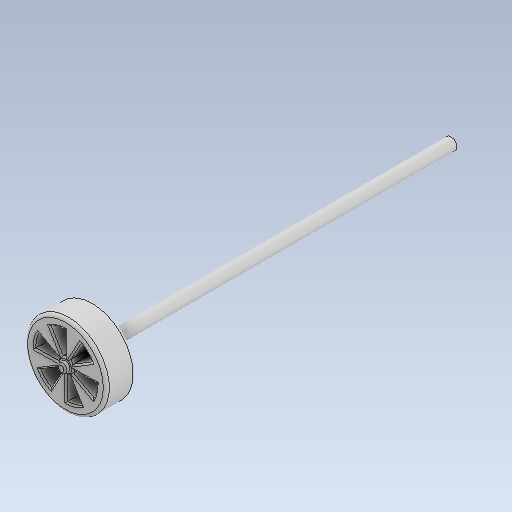
# Autodesk Inventor part: WHEEL 2_CPY1
Saved by Autodesk Inventor 2021 (Build 250183000, 183)
## iProperties
Created: 2021-07-08
Part Number: WHEEL 2_CPY1
Material: Generic
Document SubType Name: Modeling
Designer: HP
Density: 1 g/cm^3
Appearance: Default
Author: AKSHATA
Autodesk Inventor part; units mm, degrees
ref_plane "YZ Plane" through (0, 0, 0) normal (1, 0, 0) x (0, 1, 0)
ref_plane "XZ Plane" through (0, 0, 0) normal (0, 1, 0) x (-1, 0, 0)
ref_plane "XY Plane" through (0, 0, 0) normal (0, 0, 1) x (1, 0, 0)
sketch "Sketch1" plane through (0, 0, 0) normal (0, 0, 1) x (1, 0, 0)
  circle A0 centre (0, 0) radius 27.5
  dimension "d0" = 55
  constraints: 1 centre point, 1 coincident
  measures "d0" diameter of A0
extrude "Extrusion1" add sketch "Sketch1" along normal blind 20
fillet "Fillet1" radius 2 2 edges at (-27.5, 0, 20) (-27.5, 0, 0)
sketch "Sketch2" plane through (0, 0, 20) normal (0, 0, 1) x (1, 0, 0)
  circle A0 centre (0, 0) radius 21
  arc A1 (4.240585, 2.649045) -> (2.408241, 4.381823) centre (0, 0) ccw
  line L0 (4.240585, 2.649045) -> (17.925722, 10.93931)
  line L1 (0, 0) -> (0.066043, 0.120165)
  line L2 (2.408241, 4.381823) -> (10.114612, 18.403658)
  dimension "d4" = 42
  dimension "d5" = 10
  constraints: 6 end point, 4 point on circle, 2 centre point, 2 coincident
  measures "d4" diameter of A0
  measures "d5" diameter of A1
extrude "Extrusion2" cut sketch "Sketch2" against normal through all contours L0 A1 L2 A0 picked at (8.789402, 12.898997)
fillet "Fillet2" radius 1 8 edges at (11.0832, 6.7942, 20) (3.4355, 3.6329, 20) (6.2614, 11.3927, 20) (14.5084, 15.1824, 20) (11.0832, 6.7942, 0) (3.4355, 3.6329, 0) (6.2614, 11.3927, 0) (14.5084, 15.1824, 0)
pattern_circular "Circular Pattern1" count 6 over 360 about axis through (0, 0, 18) along (0, 0, 1) of "Fillet2", "Extrusion2"
sketch "Sketch3" plane through (0, 0, 20) normal (0, 0, 1) x (1, 0, 0)
  circle A0 centre (0, 0) radius 3
  dimension "d13" = 6
  constraints: 1 centre point, 1 coincident
  measures "d13" diameter of A0
extrude "Extrusion3" add sketch "Sketch3" along normal blind 3
fillet "Fillet3" radius 1 1 edges at (-3, 0, 23)
sketch "Sketch4" plane through (0, 0, 23) normal (0, 0, 1) x (1, 0, 0)
  point P0 (0, 0)
hole "Hole1" at (0, 0, 23) direction (0, 0, -1) diameter 4 end through all
sketch "Sketch5" plane through (0, 0, 20) normal (0, 0, 1) x (1, 0, 0)
  line L0 (-2.960467, 2.689913) -> (-18.814108, 11.403041)
  circle A0 centre (0, 0) radius 4
  circle A1 centre (0, 0) radius 3
  constraints: 2 coincident, 1 centre point, 3 other
extrude "Extrusion4" cut sketch "Sketch5" against normal blind 260 contours A0 | A1
sketch "Sketch6" plane through (0, 0, 20) normal (0, 0, 1) x (1, 0, 0)
  line L0 (-0.989051, -3.875794) -> (-9.708943, -19.741743)
  circle A0 centre (0, 0) radius 4
  constraints: 1 coincident, 3 other
extrude "Extrusion5" add sketch "Sketch6" against normal blind 260
body "Solid1"
